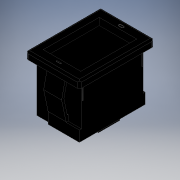
# Autodesk Inventor part: CWSB-body
Saved by Autodesk Inventor 2019 (Build 230136000, 136)
## iProperties
Created: 2024-03-12
Part Number: CWSB-body
Material: Generic
Catalog Web Link: www.cadenas.de
Description: CWSB - Miniature Power Rockers -body-
Vendor: NKKSWITCHES
Document SubType Name: Modeling
Designer: psAdmin
Manufacturer: NKKSWITCHES
Mass: 3.57429 g
Surface Area: 21.3174 cm^2
Volume: 3.57429 cm^3
Density: 1 g/cm^3
Appearance: PSOLRGB-0-0-0
Category: PARTsolutions
Company: NKKSWITCHES
Title: CWSB-body
Author: Cadenas PARTsolutions
PSOL_IDENT_0: {$CADENAS_DATA/23d-libs/nkkswitches/rocker/cw_nonillumin/parts/cwsb_body.prj},188 {VTYP=3D},{NB=CWSB
PSOL_IDENT_1: -body},{LINA=CWSB-body},{NN=CWSB - Miniature Power Rockers -body},{DATE=09.02.2024 16:13:46},{GEOMDA
PSOL_IDENT_2: TE=06.02.2009 08:16:00},{VERSION=},{LINEID=10},{WBVAR=},{WBNUMERIC=}  {NB=CWSB-body},{LINA=CWSB-body
PSOL_IDENT_3: },{KT=DUMMY},{PN=CWSB},{SRS=CWSB}
NB: CWSB-body
NN: CWSB - Miniature Power Rockers -body
NBSYN: $PN.-body
LINA: CWSB-body
CATALOG: NKK Switches
PN: CWSB
SRS: CWSB
SUPPLIER: NKKSWITCHES
ARTICLENO: CWSB-body
BOMINFO: CWSB-body
CREATOR: CADENAS GmbH
Autodesk Inventor part; units mm, degrees
sketch "Sketch_7" plane through (0, 0, 0) normal (0, 1, 0) x (-1, 0, 0)
  arc A0 (7.5438, 9.9187) -> (6.9088, 10.5537) centre (6.9088, 9.9187) ccw
  line L0 (6.9088, 10.5537) -> (-6.9088, 10.5537)
  arc A1 (-6.9088, 10.5537) -> (-7.5438, 9.9187) centre (-6.9088, 9.9187) ccw
  line L1 (-7.5438, 9.9187) -> (-7.5438, -9.9187)
  arc A2 (-7.5438, -9.9187) -> (-6.9088, -10.5537) centre (-6.9088, -9.9187) ccw
  line L2 (-6.9088, -10.5537) -> (6.9088, -10.5537)
  arc A3 (6.9088, -10.5537) -> (7.5438, -9.9187) centre (6.9088, -9.9187) ccw
  line L3 (7.5438, -9.9187) -> (7.5438, 9.9187)
  line L4 (5.2959, -7.8994) -> (5.2959, 7.8994)
  line L5 (5.2959, 7.8994) -> (-5.2959, 7.8994)
  line L6 (-5.2959, 7.8994) -> (-5.2959, -7.8994)
  line L7 (-5.2959, -7.8994) -> (5.2959, -7.8994)
  constraints: 16 end point, 8 point on circle, 4 centre point
extrude "Extrusion1" add sketch "Sketch_7" along normal blind 2.0066
sketch "Sketch_8" plane through (0, 0, 0) normal (0, 0, 1) x (1, 0, 0)
  line L0 (-8.0518, 2.5146) -> (-8.0518, 0)
  line L1 (-8.0518, 0) -> (-7.5438, 0)
  line L2 (-7.5438, 0) -> (-7.5438, 1.4986)
  arc A0 (-7.0358, 2.0066) -> (-7.5438, 1.4986) centre (-7.0358, 1.4986) ccw
  line L3 (-7.0358, 2.0066) -> (7.0358, 2.0066)
  arc A1 (7.5438, 1.4986) -> (7.0358, 2.0066) centre (7.0358, 1.4986) ccw
  line L4 (7.5438, 1.4986) -> (7.5438, 0)
  line L5 (7.5438, 0) -> (8.0518, 0)
  line L6 (8.0518, 0) -> (8.0518, 2.5146)
  line L7 (8.0518, 2.5146) -> (-8.0518, 2.5146)
  constraints: 16 end point, 4 point on circle, 2 centre point
extrude "Extrusion2" cut sketch "Sketch_8" along normal mid plane 30.48
sketch "Sketch_9" plane through (0, 0, 0) normal (1, 0, 0) x (0, 1, 0)
  line L0 (2.5146, 11.0617) -> (0, 11.0617)
  line L1 (0, 11.0617) -> (0, 10.5537)
  line L2 (0, 10.5537) -> (1.4986, 10.5537)
  arc A0 (2.0066, 10.0457) -> (1.4986, 10.5537) centre (1.4986, 10.0457) ccw
  line L3 (2.0066, 10.0457) -> (2.0066, -10.0457)
  arc A1 (1.4986, -10.5537) -> (2.0066, -10.0457) centre (1.4986, -10.0457) ccw
  line L4 (1.4986, -10.5537) -> (0, -10.5537)
  line L5 (0, -10.5537) -> (0, -11.0617)
  line L6 (0, -11.0617) -> (2.5146, -11.0617)
  line L7 (2.5146, -11.0617) -> (2.5146, 11.0617)
  constraints: 16 end point, 4 point on circle, 2 centre point
extrude "Extrusion3" cut sketch "Sketch_9" along normal mid plane 30.48
sketch "Sketch_6" plane through (0, 0, 0) normal (0, 1, 0) x (-1, 0, 0)
  line L0 (6.4516, 8.2804) -> (6.4516, 8.5344)
  line L1 (6.4516, 8.5344) -> (6.2992, 8.5344)
  line L2 (6.2992, 8.5344) -> (6.2992, 8.6995)
  line L3 (6.2992, 8.6995) -> (-6.2992, 8.6995)
  line L4 (-6.2992, 8.6995) -> (-6.2992, 8.5344)
  line L5 (-6.2992, 8.5344) -> (-6.4516, 8.5344)
  line L6 (-6.4516, 8.5344) -> (-6.4516, 8.2804)
  line L7 (-6.4516, 8.2804) -> (-6.2992, 8.2804)
  line L8 (-6.2992, 8.2804) -> (-6.2992, -8.2804)
  line L9 (-6.2992, -8.2804) -> (-6.4516, -8.2804)
  line L10 (-6.4516, -8.2804) -> (-6.4516, -8.5344)
  line L11 (-6.4516, -8.5344) -> (-6.2992, -8.5344)
  line L12 (-6.2992, -8.5344) -> (-6.2992, -8.6995)
  line L13 (-6.2992, -8.6995) -> (6.2992, -8.6995)
  line L14 (6.2992, -8.6995) -> (6.2992, -8.5344)
  line L15 (6.2992, -8.5344) -> (6.4516, -8.5344)
  line L16 (6.4516, -8.5344) -> (6.4516, -8.2804)
  line L17 (6.4516, -8.2804) -> (6.2992, -8.2804)
  line L18 (6.2992, -8.2804) -> (6.2992, 8.2804)
  line L19 (6.2992, 8.2804) -> (6.4516, 8.2804)
  constraints: 40 end point
extrude "Extrusion4" add sketch "Sketch_6" against normal blind 15.1892
sketch "Sketch_1" plane through (0, -14.1986, 0) normal (0, 1, 0) x (1, 0, 0)
  line L0 (-6.4516, -8.2804) -> (-6.4516, -8.5344)
  line L1 (-6.4516, -8.5344) -> (-6.2992, -8.5344)
  line L2 (-6.2992, -8.5344) -> (-6.2992, -8.6995)
  line L3 (-6.2992, -8.6995) -> (-2.286, -8.6995)
  line L4 (-2.286, -8.6995) -> (-2.286, -9.2964)
  line L5 (-2.286, -9.2964) -> (6.2992, -9.2964)
  line L6 (6.2992, -9.2964) -> (6.2992, -8.5344)
  line L7 (6.2992, -8.5344) -> (6.4516, -8.5344)
  line L8 (6.4516, -8.5344) -> (6.4516, -8.2804)
  line L9 (6.4516, -8.2804) -> (6.2992, -8.2804)
  line L10 (6.2992, -8.2804) -> (6.2992, 8.2804)
  line L11 (6.2992, 8.2804) -> (6.4516, 8.2804)
  line L12 (6.4516, 8.2804) -> (6.4516, 8.5344)
  line L13 (6.4516, 8.5344) -> (6.2992, 8.5344)
  line L14 (6.2992, 8.5344) -> (6.2992, 9.2964)
  line L15 (6.2992, 9.2964) -> (-2.286, 9.2964)
  line L16 (-2.286, 9.2964) -> (-2.286, 8.6995)
  line L17 (-2.286, 8.6995) -> (-6.2992, 8.6995)
  line L18 (-6.2992, 8.6995) -> (-6.2992, 8.5344)
  line L19 (-6.2992, 8.5344) -> (-6.4516, 8.5344)
  line L20 (-6.4516, 8.5344) -> (-6.4516, 8.2804)
  line L21 (-6.4516, 8.2804) -> (-6.2992, 8.2804)
  line L22 (-6.2992, 8.2804) -> (-6.2992, -8.2804)
  line L23 (-6.2992, -8.2804) -> (-6.4516, -8.2804)
  constraints: 48 end point
extrude "Extrusion5" add sketch "Sketch_1" along normal blind 3.0226
sketch "Sketch_10" plane through (0, 0, 0) normal (1, 0, 0) x (0, 1, 0)
  line L0 (-5.08, 10.5537) -> (-11.0341, 9.2964)
  line L1 (-11.0341, 9.2964) -> (-14.1986, 9.2964)
  line L2 (-14.1986, 9.2964) -> (-14.1986, -9.2964)
  line L3 (-14.1986, -9.2964) -> (-11.0341, -9.2964)
  line L4 (-11.0341, -9.2964) -> (-5.08, -10.5537)
  line L5 (-5.08, -10.5537) -> (0, -9.4488)
  line L6 (0, -9.4488) -> (0, -8.799)
  line L7 (0, -8.799) -> (-5.082, -9.9043)
  line L8 (-5.082, -9.9043) -> (-9.3489, -9.0033)
  arc A0 (-9.5504, -8.7547) -> (-9.3489, -9.0033) centre (-9.2964, -8.7547) ccw
  line L9 (-9.5504, -8.7547) -> (-9.5504, -8.6995)
  line L10 (-9.5504, -8.6995) -> (0, -8.6995)
  line L11 (0, -8.6995) -> (0, 8.6995)
  line L12 (0, 8.6995) -> (-9.5504, 8.6995)
  line L13 (-9.5504, 8.6995) -> (-9.5504, 8.7547)
  arc A1 (-9.3489, 9.0033) -> (-9.5504, 8.7547) centre (-9.2964, 8.7547) ccw
  line L14 (-9.3489, 9.0033) -> (-5.082, 9.9043)
  line L15 (-5.082, 9.9043) -> (0, 8.799)
  line L16 (0, 8.799) -> (0, 9.4488)
  line L17 (0, 9.4488) -> (-5.08, 10.5537)
  constraints: 36 end point, 4 point on circle, 2 centre point
extrude "Extrusion6" add sketch "Sketch_10" along normal mid plane 5.08
sketch "Sketch_13" plane through (0, 0, 0) normal (0, 0, 1) x (1, 0, 0)
  line L0 (-6.4516, -16.5862) -> (6.4516, -16.5862)
  line L1 (6.4516, -16.5862) -> (6.4516, -4.318)
  line L2 (6.4516, -4.318) -> (6.2992, -4.318)
  line L3 (6.2992, -4.318) -> (6.2992, -16.2052)
  line L4 (6.2992, -16.2052) -> (-6.2992, -16.2052)
  line L5 (-6.2992, -16.2052) -> (-6.2992, -4.318)
  line L6 (-6.2992, -4.318) -> (-6.4516, -4.318)
  line L7 (-6.4516, -4.318) -> (-6.4516, -16.5862)
  constraints: 16 end point
extrude "Extrusion7" cut sketch "Sketch_13" along normal mid plane 25.4
sketch "Sketch_2" plane through (0, 0, 0) normal (0, 1, 0) x (-1, 0, 0)
  arc A0 (0.381, -9.1631) -> (0.381, -8.5026) centre (0.381, -8.8329) ccw
  line L0 (0.381, -8.5026) -> (-0.381, -8.5026)
  arc A1 (-0.381, -8.5026) -> (-0.381, -9.1631) centre (-0.381, -8.8329) ccw
  line L1 (-0.381, -9.1631) -> (0.381, -9.1631)
  arc A2 (0.381, -9.0869) -> (0.381, -8.5788) centre (0.381, -8.8329) ccw
  line L2 (0.381, -8.5788) -> (-0.381, -8.5788)
  arc A3 (-0.381, -8.5788) -> (-0.381, -9.0869) centre (-0.381, -8.8329) ccw
  line L3 (-0.381, -9.0869) -> (0.381, -9.0869)
  constraints: 8 end point, 8 point on circle, 4 centre point
extrude "Extrusion8" add sketch "Sketch_2" along normal blind 2.0828
sketch "Sketch_3" plane through (0, 0, 0) normal (0, 1, 0) x (-1, 0, 0)
  line L0 (0.635, 8.7058) -> (0.635, 8.9598)
  line L1 (0.635, 8.9598) -> (-0.635, 8.9598)
  line L2 (-0.635, 8.9598) -> (-0.635, 8.7058)
  line L3 (-0.635, 8.7058) -> (0.635, 8.7058)
  constraints: 8 end point
extrude "Extrusion9" add sketch "Sketch_3" along normal blind 2.0828
sketch "Sketch_12" plane through (0, -14.1986, 0) normal (0, 1, 0) x (1, 0, 0)
  line L0 (-8.7897, 13.35) -> (-8.7897, -12.337)
  line L1 (-8.7897, -12.337) -> (9.6509, -12.337)
  line L2 (9.6509, -12.337) -> (9.6509, 13.35)
  line L3 (9.6509, 13.35) -> (-8.7897, 13.35)
  arc A0 (2.8067, -6.8961) -> (3.0607, -7.1501) centre (3.0607, -6.8961) ccw
  line L4 (3.0607, -7.1501) -> (4.9149, -7.1501)
  arc A1 (4.9149, -7.1501) -> (5.1689, -6.8961) centre (4.9149, -6.8961) ccw
  line L5 (5.1689, -6.8961) -> (5.1689, -5.0419)
  arc A2 (5.1689, -5.0419) -> (4.9149, -4.7879) centre (4.9149, -5.0419) ccw
  line L6 (4.9149, -4.7879) -> (4.3815, -4.7879)
  line L7 (4.3815, -4.7879) -> (4.3815, -6.3627)
  line L8 (4.3815, -6.3627) -> (3.5941, -6.3627)
  line L9 (3.5941, -6.3627) -> (3.5941, -4.7879)
  line L10 (3.5941, -4.7879) -> (3.0607, -4.7879)
  arc A3 (3.0607, -4.7879) -> (2.8067, -5.0419) centre (3.0607, -5.0419) ccw
  line L11 (2.8067, -5.0419) -> (2.8067, -6.8961)
  arc A4 (1.3081, 6.0579) -> (1.5621, 5.8039) centre (1.5621, 6.0579) ccw
  line L12 (1.5621, 5.8039) -> (2.0955, 5.8039)
  line L13 (2.0955, 5.8039) -> (2.0955, 7.3787)
  line L14 (2.0955, 7.3787) -> (2.8829, 7.3787)
  line L15 (2.8829, 7.3787) -> (2.8829, 5.8039)
  line L16 (2.8829, 5.8039) -> (3.4163, 5.8039)
  arc A5 (3.4163, 5.8039) -> (3.6703, 6.0579) centre (3.4163, 6.0579) ccw
  line L17 (3.6703, 6.0579) -> (3.6703, 7.9121)
  arc A6 (3.6703, 7.9121) -> (3.4163, 8.1661) centre (3.4163, 7.9121) ccw
  line L18 (3.4163, 8.1661) -> (1.5621, 8.1661)
  arc A7 (1.5621, 8.1661) -> (1.3081, 7.9121) centre (1.5621, 7.9121) ccw
  line L19 (1.3081, 7.9121) -> (1.3081, 6.0579)
  arc A8 (1.3081, 2.0955) -> (1.5621, 1.8415) centre (1.5621, 2.0955) ccw
  line L20 (1.5621, 1.8415) -> (3.4163, 1.8415)
  arc A9 (3.4163, 1.8415) -> (3.6703, 2.0955) centre (3.4163, 2.0955) ccw
  line L21 (3.6703, 2.0955) -> (3.6703, 3.9497)
  arc A10 (3.6703, 3.9497) -> (3.4163, 4.2037) centre (3.4163, 3.9497) ccw
  line L22 (3.4163, 4.2037) -> (2.8829, 4.2037)
  line L23 (2.8829, 4.2037) -> (2.8829, 2.6289)
  line L24 (2.8829, 2.6289) -> (2.0955, 2.6289)
  line L25 (2.0955, 2.6289) -> (2.0955, 4.2037)
  line L26 (2.0955, 4.2037) -> (1.5621, 4.2037)
  arc A11 (1.5621, 4.2037) -> (1.3081, 3.9497) centre (1.5621, 3.9497) ccw
  line L27 (1.3081, 3.9497) -> (1.3081, 2.0955)
  arc A12 (-3.6703, 2.0955) -> (-3.4163, 1.8415) centre (-3.4163, 2.0955) ccw
  line L28 (-3.4163, 1.8415) -> (-1.5621, 1.8415)
  arc A13 (-1.5621, 1.8415) -> (-1.3081, 2.0955) centre (-1.5621, 2.0955) ccw
  line L29 (-1.3081, 2.0955) -> (-1.3081, 3.9497)
  arc A14 (-1.3081, 3.9497) -> (-1.5621, 4.2037) centre (-1.5621, 3.9497) ccw
  line L30 (-1.5621, 4.2037) -> (-2.0955, 4.2037)
  line L31 (-2.0955, 4.2037) -> (-2.0955, 2.6289)
  line L32 (-2.0955, 2.6289) -> (-2.8829, 2.6289)
  line L33 (-2.8829, 2.6289) -> (-2.8829, 4.2037)
  line L34 (-2.8829, 4.2037) -> (-3.4163, 4.2037)
  arc A15 (-3.4163, 4.2037) -> (-3.6703, 3.9497) centre (-3.4163, 3.9497) ccw
  line L35 (-3.6703, 3.9497) -> (-3.6703, 2.0955)
  line L36 (-3.6703, 7.9121) -> (-3.6703, 6.0579)
  arc A16 (-3.6703, 6.0579) -> (-3.4163, 5.8039) centre (-3.4163, 6.0579) ccw
  line L37 (-3.4163, 5.8039) -> (-2.8829, 5.8039)
  line L38 (-2.8829, 5.8039) -> (-2.8829, 7.3787)
  line L39 (-2.8829, 7.3787) -> (-2.0955, 7.3787)
  line L40 (-2.0955, 7.3787) -> (-2.0955, 5.8039)
  line L41 (-2.0955, 5.8039) -> (-1.5621, 5.8039)
  arc A17 (-1.5621, 5.8039) -> (-1.3081, 6.0579) centre (-1.5621, 6.0579) ccw
  line L42 (-1.3081, 6.0579) -> (-1.3081, 7.9121)
  arc A18 (-1.3081, 7.9121) -> (-1.5621, 8.1661) centre (-1.5621, 7.9121) ccw
  line L43 (-1.5621, 8.1661) -> (-3.4163, 8.1661)
  arc A19 (-3.4163, 8.1661) -> (-3.6703, 7.9121) centre (-3.4163, 7.9121) ccw
  arc A20 (-5.1689, -6.8961) -> (-4.9149, -7.1501) centre (-4.9149, -6.8961) ccw
  line L44 (-4.9149, -7.1501) -> (-3.0607, -7.1501)
  arc A21 (-3.0607, -7.1501) -> (-2.8067, -6.8961) centre (-3.0607, -6.8961) ccw
  line L45 (-2.8067, -6.8961) -> (-2.8067, -5.0419)
  arc A22 (-2.8067, -5.0419) -> (-3.0607, -4.7879) centre (-3.0607, -5.0419) ccw
  line L46 (-3.0607, -4.7879) -> (-3.5941, -4.7879)
  line L47 (-3.5941, -4.7879) -> (-3.5941, -6.3627)
  line L48 (-3.5941, -6.3627) -> (-4.3815, -6.3627)
  line L49 (-4.3815, -6.3627) -> (-4.3815, -4.7879)
  line L50 (-4.3815, -4.7879) -> (-4.9149, -4.7879)
  arc A23 (-4.9149, -4.7879) -> (-5.1689, -5.0419) centre (-4.9149, -5.0419) ccw
  line L51 (-5.1689, -5.0419) -> (-5.1689, -6.8961)
  constraints: 104 end point, 48 point on circle, 24 centre point
extrude "Extrusion10" cut sketch "Sketch_12" against normal blind 0.9906
sketch "Sketch_4" plane through (0, -14.1986, 0) normal (0, 1, 0) x (1, 0, 0)
  line L0 (-0.3937, 1.9558) -> (0.3937, 1.9558)
  line L1 (0.3937, 1.9558) -> (0.3937, 8.0518)
  line L2 (0.3937, 8.0518) -> (-0.3937, 8.0518)
  line L3 (-0.3937, 8.0518) -> (-0.3937, 1.9558)
  constraints: 8 end point
extrude "Extrusion11" add sketch "Sketch_4" against normal blind 6.223
ref_plane "to_dummy_XY" through (0, 0, 0) normal (0, -1, 0) x (1, 0, 0)
ref_plane "to_dummy_YZ" through (0, 0, 0) normal (1, 0, 0) x (0, 0, 1)
ref_plane "to_dummy_ZX" through (0, 0, 0) normal (0, 0, 1) x (0, -1, 0)
ref_plane "to_rocker_XY" through (0, 0, 0) normal (0, -1, 0) x (1, 0, 0)
ref_plane "to_rocker_YZ" through (0, 0, 0) normal (1, 0, 0) x (0, 0, 1)
ref_plane "to_rocker_ZX" through (0, 0, 0) normal (0, 0, 1) x (0, -1, 0)
ref_plane "to_terminals_XY" through (0, -14.0462, 0) normal (0, 1, 0) x (1, 0, 0)
ref_plane "to_terminals_YZ" through (0, -14.0462, 0) normal (1, 0, 0) x (0, 0, -1)
ref_plane "to_terminals_ZX" through (0, -14.0462, 0) normal (0, 0, -1) x (0, 1, 0)
body "Solid1"
